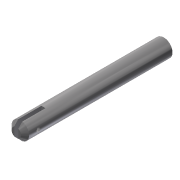
# Autodesk Inventor part: LIVER SHAFT
Saved by Autodesk Inventor 2014 (Build 180170000, 170)
## iProperties
Created: 2014-12-18
Part Number: LIVER SHAFT
Material: Steel, Alloy
Document SubType Name: Modeling
Designer: Ebrahim
Density: 7.85 g/cm^3
Appearance: Semi-Polished
Mass: 105.947 g
Surface Area: 50.7442 cm^2
Volume: 13.4965 cm^3
Author: Ebrahim
Autodesk Inventor part; units mm, degrees
ref_plane "YZ Plane" through (0, 0, 0) normal (1, 0, 0) x (0, 1, 0)
ref_plane "XZ Plane" through (0, 0, 0) normal (0, 1, 0) x (-1, 0, 0)
ref_plane "XY Plane" through (0, 0, 0) normal (0, 0, 1) x (1, 0, 0)
sketch "Sketch1" plane through (0, 0, 0) normal (0, 1, 0) x (-1, 0, 0)
  circle A0 centre (0, 0) radius 6.5
  dimension "d0" = 13
  constraints: 1 centre point, 1 coincident
  measures "d0" diameter of A0
extrude "Extrusion1" add sketch "Sketch1" along normal blind 109
chamfer "Chamfer1" distance 3 angle 45 1 edges at (6.5, 0, 0)
sketch "Sketch2" plane through (0, 0, 0) normal (1, 0, 0) x (0, 1, 0)
  line L0 (20, 11.2856) -> (-12.0513, 11.2856)
  line L1 (-12.0513, 11.2856) -> (-12.0513, -8.7625)
  line L2 (-12.0513, -8.7625) -> (20, -8.7625)
  line L3 (20, -8.7625) -> (20, 11.2856)
  line L4 (109, -6.5) -> (109, 6.5) construction
  line L5 (3, 6.5) -> (3, -6.5) construction
  line L6 (0, -3.5) -> (0, 3.5) construction
  point P0 (0, 0)
  dimension "d6" = 20
  constraints: 8 end point, 2 parallel, 1 horizontal, 1 perpendicular
  measures "d6" distance between parallel lines of L3 L6
extrude "Extrusion2" cut sketch "Sketch2" along normal mid plane 3
sketch "Sketch3" plane through (0, 0, 0) normal (1, 0, 0) x (0, 1, 0)
  line L0 (-21.8, 0) -> (130.8, 0) construction
  line L1 (0, -3.1623) -> (0, 3.1623) construction
  point P0 (0, 0)
  point P1 (10, 0)
  dimension "d9" = 10
  constraints: 1 point on line
  measures "d9" distance from line of point (10, 0) L1
hole "Hole1" at (0, 10, 0) direction (1, 0, 0) diameter 3 end through all
mirror "Mirror1" about plane through (0, 0, 0) normal (1, 0, 0) of "Hole1"
body "Solid1"
